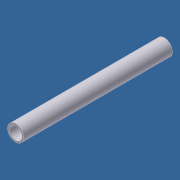
# Autodesk Inventor part: FE-00006-06
Saved by Autodesk Inventor 2012 (Build 160160000, 160)
## iProperties
Created: 2008-05-25
Part Number: FE-00006-06
Document SubType Name: Modeling
Designer: firstuser
Density: 1 g/cm^3
Mass: 101.737 g
Surface Area: 576.909 cm^2
Volume: 101.737 cm^3
Material: Default
Author: firstuser
Autodesk Inventor part; units mm, degrees
ref_plane "XZ Plane" through (0, 0, 0) normal (0, 1, 0) x (-1, 0, 0)
ref_plane "XY Plane" through (0, 0, 0) normal (0, 0, 1) x (1, 0, 0)
sketch "Sketch1" plane through (0, 0, 0) normal (0, 0, 1) x (1, 0, 0)
  circle A0 centre (0, 0) radius 16.6688
  circle A1 centre (0, 0) radius 13.0969
  dimension "d0" = 33.3375
  dimension "d1" = 26.1938
  constraints: 2 centre point, 1 coincident
  measures "d0" diameter of A0
  measures "d1" diameter of A1
extrude "Extrusion1" add sketch "Sketch1" along normal blind 304.8
ref_plane "Work Plane1" through (0, 0, 0) normal (1, 0, 0) x (0, 0, 1)
sketch "Sketch2" plane through (0, 0, 0) normal (1, 0, 0) x (0, 0, 1)
  line L0 (0, -16.6688) -> (304.8, -16.6688) projected
  line L1 (0, 16.6688) -> (304.8, 16.6688) projected
  line L2 (304.8, 13.0969) -> (304.8, -13.0969) projected
  line L3 (304.8, 16.6688) -> (304.8, -16.6688) projected
  circle A0 centre (165.1, 0) radius 3.175
  circle A1 centre (165.1, 0) radius 2.5527
  line L4 (-60.96, 0) -> (365.76, 0) projected
  dimension "d5" = 6.35
  dimension "d6" = 5.1054
  dimension "d7" = 139.7
  constraints: 2 centre point, 1 coincident, 1 point on line
  measures "d5" diameter of A0
  measures "d6" diameter of A1
  measures "d7" distance from line of A0.centre L2
extrude "Extrusion2" cut sketch "Sketch2" against normal blind 304.8 contours L4 A1 | A1 L4
thread "Thread1" size "1/4-28 UNF" class "2B" standard "ANSI Unified Screw Threads" full length
body "Solid1"
